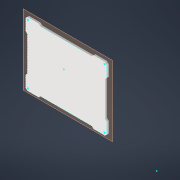
# Autodesk Inventor part: Lid
Saved by Autodesk Inventor 2021.1 (Build 251245010, 245A)
## iProperties
Created: 2020-11-27
Part Number: Lid
Material: Generic
Document SubType Name: Modeling
Designer: Alex
Density: 1 g/cm^3
Appearance: Default
Author: Alex
Autodesk Inventor part; units mm, degrees
ref_plane "YZ Plane" through (0, 0, 0) normal (1, 0, 0) x (0, 1, 0)
ref_plane "XZ Plane" through (0, 0, 0) normal (0, 1, 0) x (-1, 0, 0)
ref_plane "XY Plane" through (0, 0, 0) normal (0, 0, 1) x (1, 0, 0)
ref_plane "Work Plane1" through (-158.3203, 64.5406, -57.1768) normal (0, 0, 1) x (1, 0, 0)
sketch "Sketch1" plane through (-158.3203, 64.5406, -57.1768) normal (0, 0, 1) x (1, 0, 0)
  circle A0 centre (67, -52) radius 2 construction
  circle A1 centre (-67, 52) radius 2 construction
  circle A2 centre (-67, -52) radius 2 construction
  circle A3 centre (67, 52) radius 2 construction
  line L0 (-71, 33) -> (-68, 30) projected
  line L1 (-68, 30) -> (-68, -30) projected
  line L2 (-68, -30) -> (-71, -33) projected
  line L3 (-71, -33) -> (-71, -53) projected
  line L4 (-71, -53) -> (-68, -56) projected
  line L5 (-68, -56) -> (-48, -56) projected
  line L6 (-48, -56) -> (-45, -53) projected
  line L7 (-45, -53) -> (45, -53) projected
  line L8 (45, -53) -> (48, -56) projected
  line L9 (48, -56) -> (68, -56) projected
  line L10 (68, -56) -> (71, -53) projected
  line L11 (71, -53) -> (71, -33) projected
  line L12 (71, -33) -> (68, -30) projected
  line L13 (68, -30) -> (68, 30) projected
  line L14 (68, 30) -> (71, 33) projected
  line L15 (71, 33) -> (71, 53) projected
  line L16 (71, 53) -> (68, 56) projected
  line L17 (68, 56) -> (48, 56) projected
  line L18 (48, 56) -> (45, 53) projected
  line L19 (45, 53) -> (-45, 53) projected
  line L20 (-45, 53) -> (-48, 56) projected
  line L21 (-48, 56) -> (-68, 56) projected
  line L22 (-68, 56) -> (-71, 53) projected
  line L23 (-71, 53) -> (-71, 33) projected
  line L24 (-65, -47) -> (-65, 39.05) construction
  line L25 (-55, 39.05) -> (-65, 39.05) construction
  line L26 (-44.05, 50) -> (-55, 39.05) construction
  line L27 (-44.05, 50) -> (44.05, 50) construction
  line L28 (55, 39.05) -> (44.05, 50) construction
  line L29 (65, 39.05) -> (55, 39.05) construction
  line L30 (65, 39.05) -> (65, -47) construction
  line L31 (65, -47) -> (62, -50) construction
  line L32 (62, -50) -> (-62, -50) construction
  line L33 (-62, -50) -> (-65, -47) construction
  point P0 (158.3203, -64.5406)
extrude "Extrusion1" add sketch "Sketch1" along normal blind 3
sketch "Sketch2" plane through (-158.3203, 64.5406, -54.1768) normal (0, 0, 1) x (1, 0, 0)
  circle A0 centre (-67, -52) radius 2 construction
  circle A1 centre (67, -52) radius 2 construction
  circle A2 centre (67, 52) radius 2 construction
  circle A3 centre (-67, 52) radius 2 construction
  point P0 (158.3203, -64.5406)
  constraints: 4 coincident
hole "Hole1" at (-225.3203, 116.5406, -54.1768) at (-91.3203, 116.5406, -54.1768) at (-91.3203, 12.5406, -54.1768) at (-225.3203, 12.5406, -54.1768) direction (0, 0, -1) diameter 3.4 depth 5 clearance for "Hex Head Cap Screw ISO 24017" size "M3" standard "ISO"
sketch "Sketch3" plane through (-158.3203, 64.5406, -54.1768) normal (0, 0, 1) x (1, 0, 0)
  circle A0 centre (-4.1, 8.7) radius 1.6 construction
  circle A1 centre (67, -52) radius 1.7 construction
  circle A2 centre (-67, 52) radius 1.7 construction
  circle A3 centre (67, 52) radius 1.7 construction
  circle A4 centre (-67, -52) radius 1.7 construction
  line L0 (-68, 30) -> (-68, -30) construction
  line L1 (-68, -30) -> (-71, -33) construction
  line L2 (-71, -33) -> (-71, -53) construction
  line L3 (-71, -53) -> (-68, -56) construction
  line L4 (-68, -56) -> (-48, -56) construction
  line L5 (-48, -56) -> (-45, -53) construction
  line L6 (-45, -53) -> (45, -53) construction
  line L7 (45, -53) -> (48, -56) construction
  line L8 (48, -56) -> (68, -56) construction
  line L9 (68, -56) -> (71, -53) construction
  line L10 (71, -53) -> (71, -33) construction
  line L11 (71, -33) -> (68, -30) construction
  line L12 (68, -30) -> (68, 30) construction
  line L13 (68, 30) -> (71, 33) construction
  line L14 (71, 33) -> (71, 53) construction
  line L15 (71, 53) -> (68, 56) construction
  line L16 (68, 56) -> (48, 56) construction
  line L17 (48, 56) -> (45, 53) construction
  line L18 (45, 53) -> (-45, 53) construction
  line L19 (-45, 53) -> (-48, 56) construction
  line L20 (-48, 56) -> (-68, 56) construction
  line L21 (-68, 56) -> (-71, 53) construction
  line L22 (-71, 53) -> (-71, 33) construction
  line L23 (-71, 33) -> (-68, 30) construction
  point P0 (158.3203, -64.5406)
body "Solid1"
